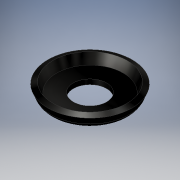
# Autodesk Inventor part: TopBushingWasher
Saved by Autodesk Inventor 2019 (Build 230136000, 136)
## iProperties
Created: 2020-12-10
Part Number: TopBushingWasher
Material: Aluminum
Document SubType Name: Modeling
Designer: Anass Hamdi
Density: 2.7 g/cm^3
Appearance: Aluminum Frame - Anodized Dark Bronze Satin
Author: Anass Hamdi
Autodesk Inventor part; units mm, degrees
ref_plane "YZ Plane" through (0, 0, 0) normal (1, 0, 0) x (0, 1, 0)
ref_plane "XZ Plane" through (0, 0, 0) normal (0, 1, 0) x (-1, 0, 0)
ref_plane "XY Plane" through (0, 0, 0) normal (0, 0, 1) x (1, 0, 0)
sketch "Sketch1" plane through (0, 0, 0) normal (0, 0, 1) x (1, 0, 0)
  line L0 (11.9, 0) -> (11.9, 3.5) construction
  line L1 (11.9, 3.5) -> (10.5, 3.5) construction
  line L2 (0, 0) -> (0, 1.4)
  line L3 (10.5, 3.5) -> (10.5, 4) construction
  line L4 (11.9, 3.5) -> (10.5, 4)
  line L5 (0, 0) -> (10.5, 0)
  line L6 (10.5, 0) -> (11.9, 3.5)
  line L7 (10.5, 4) -> (9.46, 1.4)
  line L8 (0, 1.4) -> (9.46, 1.4)
  dimension "d0" = 11.9
  dimension "d1" = 3.5
  dimension "d2" = 1.4
  dimension "d3" = 0.5
  dimension "d4" = 1.4
  constraints: 18 end point, 3 horizontal, 2 vertical, 1 parallel
  measures "d0" distance of L2.start L0.start
  measures "d1" distance of L0.start L0.end
  measures "d2" distance of L0.end L1.end
  measures "d3" distance of L1.end L3.end
  measures "d4" distance of L2.start L2.end
revolve "Revolution1" add sketch "Sketch1" angle 360 about axis through (0, 0, 0) along (0, 1, 0)
sketch "Sketch2" plane through (0, 1.4, 0) normal (0, 1, 0) x (1, 0, 0)
  circle A0 centre (0, 0) radius 4.7
  dimension "d6" = 9.4
  constraints: 1 centre point, 1 coincident
  measures "d6" diameter of A0
extrude "Extrusion1" cut sketch "Sketch2" against normal through all
fillet "Fillet1" radius 2.4 1 edges at (-10.5, 0, 0)
body "Solid1"
